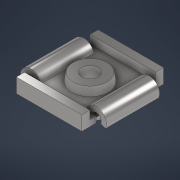
# Autodesk Inventor part: 18102021-002-06
Saved by Autodesk Inventor 2021 (Build 250183000, 183)
## iProperties
Created: 2021-10-15
Part Number: 18102021-002-06
Material: Stainless Steel
Document SubType Name: Modeling
Designer: DuctopwH
Density: 8 g/cm^3
Appearance: Semi-Polished
Author: DuctopwH
Autodesk Inventor part; units mm, degrees
ref_plane "YZ Plane" through (0, 0, 0) normal (1, 0, 0) x (0, 1, 0)
ref_plane "XZ Plane" through (0, 0, 0) normal (0, 1, 0) x (-1, 0, 0)
ref_plane "XY Plane" through (0, 0, 0) normal (0, 0, 1) x (1, 0, 0)
sketch "Sketch2" plane through (0, 0, 0) normal (0, 0, 1) x (1, 0, 0)
  line L0 (0, 0) -> (0, 8.3073) construction
  line L1 (2, 0) -> (2, 7.5)
  line L2 (2, 7.5) -> (4.1473, 7.5)
  line L3 (4.1473, 7.5) -> (4.5, 5.5)
  line L4 (4.5, 5.5) -> (4.5, 4)
  line L5 (4.5, 4) -> (4, 4)
  line L6 (4, 4) -> (4, 0)
  line L7 (4, 0) -> (2, 0)
  dimension "d1" = 4
  dimension "d2" = 7.5
  dimension "d3" = 3.5
  dimension "d4" = 10
  dimension "d5" = 8
  dimension "d6" = 9
  dimension "d7" = 2
  constraints: 16 end point, 4 perpendicular, 2 vertical, 1 parallel, 1 point on line
  measures "d1" diameter of L1 L0
  measures "d2" distance between parallel lines of L7 L2
  measures "d3" distance between parallel lines of L5 L2
  measures "d4" angle of L0 L3
  measures "d5" diameter of L6 L0
  measures "d6" diameter of L3.end L0
  measures "d7" distance from line of L3.end L2
revolve "Revolution1" add sketch "Sketch2" angle 360 about axis through (0, 0, 0) along (0, 1, 0)
sketch "Sketch3" plane through (0, 0, 0) normal (0, 0, 1) x (1, 0, 0)
  line L0 (0, 0) -> (0, 7.5)
  line L1 (-4.1473, 7.5) -> (4.1473, 7.5) projected
  circle A0 centre (-8, 5) radius 1.25
  circle A1 centre (-8, 5) radius 2.5
  line L2 (-4.5, 4) -> (4.5, 4) projected
  line L3 (-7.25, 4) -> (-4.5, 4)
  line L4 (-4.5, 5.5) -> (-4.5, 4) projected
  line L5 (-4.5, 5.5) -> (-5.5505, 5.5)
  circle A2 centre (8, 5) radius 1.25
  circle A3 centre (8, 5) radius 2.5
  line L6 (7.25, 4) -> (4.5, 4)
  line L7 (4.5, 5.5) -> (5.5505, 5.5)
  line L8 (-10.2913, 4) -> (-9.1121, 4.4292)
  line L9 (-8, 5) -> (-8, -2.6119) construction
  line L10 (-4.5, 5.5) -> (-2.8248, 5.5)
  line L11 (-4.5, 5.5) -> (4.5, 5.5) projected
  line L12 (-2.8248, 4) -> (-2.8248, 5.5)
  line L13 (4.5, 5.5) -> (2.7431, 5.5)
  line L14 (2.7431, 5.5) -> (2.7431, 4)
  line L15 (10.2913, 4) -> (9.1121, 4.4292)
  line L16 (-6.75, 5) -> (-6.75, 4)
  line L17 (6.75, 5) -> (6.75, 4)
  dimension "d9" = 5
  dimension "d10" = 2.5
  dimension "d11" = 16
  dimension "d12" = 70
  constraints: 28 end point, 8 symmetric about line, 7 point on circle, 7 point on line, 5 perpendicular, 3 centre point, 3 tangent, 2 coincident, 1 horizontal, 1 midpoint, 1 vertical, 5 other
  measures "d9" diameter of A1
  measures "d10" diameter of A0
  measures "d11" distance of point (8, 5) A0.centre
  measures "d12" angle of L8 L9
extrude "Extrusion1" add sketch "Sketch3" along normal mid plane 13 contours L2 L4 L10 L12 | L14 L11 L7 A3 L6 L2 | L3 A1 L5 L4 | L3 L16 A0 L8 A1 | A3 L15 A2 L17 L6
sketch "Sketch4" plane through (2.7431, 4, -6.5) normal (0, -1, 0) x (1, 0, 0)
  line L0 (-9.4931, 0) -> (-9.4931, 13) projected
  line L1 (4.0069, 13) -> (4.0069, 0) projected
  line L2 (5.2569, -3.5) -> (-10.7431, -3.5)
  line L3 (-2.7431, -3.5) -> (-2.7431, 6.5)
  line L4 (5.2569, -3.5) -> (5.2569, 0)
  line L5 (0, 0) -> (2.8074, 0) projected
  line L6 (5.2569, 0) -> (0, 0)
  line L7 (0, 0) -> (0, 2.8945)
  arc A0 (-5.5678, 2.997) -> (0, 2.9327) centre (-2.7431, 6.5) ccw projected
  line L8 (-10.7431, -3.5) -> (-10.7431, 0)
  line L9 (-8.2936, 0) -> (-5.5678, 0) projected
  line L10 (-10.7431, 0) -> (-5.5678, 0)
  line L11 (-5.5678, 0) -> (-5.5678, 2.997) projected
  line L12 (-5.5678, 0) -> (-5.5678, 2.997)
  line L13 (-2.7431, 6.5) -> (4.0069, 6.5)
  line L14 (5.2569, 16.5) -> (-10.7431, 16.5)
  line L15 (5.2569, 16.5) -> (5.2569, 13)
  line L16 (0, 13) -> (2.8074, 13)
  line L17 (5.2569, 13) -> (0, 13)
  line L18 (0, 13) -> (0, 10.1055)
  arc A1 (0, 10.0673) -> (-5.5678, 10.003) centre (-2.7431, 6.5) ccw
  line L19 (-10.7431, 16.5) -> (-10.7431, 13)
  line L20 (-8.2936, 13) -> (-5.5678, 13)
  line L21 (-10.7431, 13) -> (-5.5678, 13)
  line L22 (-5.5678, 13) -> (-5.5678, 10.003)
  line L23 (-5.5678, 13) -> (-5.5678, 10.003)
  arc A2 (0, 2.9327) -> (0, 10.0673) centre (-2.7431, 6.5) ccw projected
  arc A3 (-5.5678, 10.003) -> (-5.5678, 2.997) centre (-2.7431, 6.5) ccw projected
  point P0 (-2.7431, 16.5)
  dimension "d15" = 16
  dimension "d21" = 20
  constraints: 38 end point, 12 symmetric about line, 3 perpendicular, 3 vertical, 2 midpoint, 2 point on circle, 1 centre point, 1 collinear, 1 other
  measures "d15" distance of L2.start L2.end
  measures "d21" distance between parallel lines of L2 L14
extrude "Extrusion2" add sketch "Sketch4" against normal up to surface (1.5 mm away) contours L10 L9 L11 A0 L3 L2 L8 | L21 L19 L14 L15 L17 L1 L13 A2 A1 L22 L20 | L3 A0 A2 L13 L1 L6 L4 L2
sketch "Sketch5" plane through (5.5505, 5.5, 6.5) normal (0, 1, 0) x (1, 0, 0)
  line L0 (-5.5505, 6.5) -> (4.9752, 6.5)
  line L1 (-13.5505, 16.5) -> (2.4495, 16.5) projected
  line L2 (2.4495, 16.5) -> (-13.5505, 16.5)
  line L3 (-13.5505, 16.5) -> (-13.5505, 14.5)
  line L4 (-13.5505, 14.5) -> (2.4495, 14.5)
  line L5 (2.4495, 14.5) -> (2.4495, 16.5)
  line L6 (-13.5505, -3.5) -> (2.4495, -3.5)
  line L7 (2.4495, -3.5) -> (-13.5505, -3.5)
  line L8 (-13.5505, -3.5) -> (-13.5505, -1.5)
  line L9 (-13.5505, -1.5) -> (2.4495, -1.5)
  line L10 (2.4495, -1.5) -> (2.4495, -3.5)
  dimension "d18" = 16
  constraints: 20 end point, 5 symmetric about line, 2 horizontal, 2 parallel, 1 perpendicular
  measures "d18" distance between parallel lines of L9 L4
extrude "Extrusion3" add sketch "Sketch5" along normal up to surface (2 mm away)
body "Solid1"
